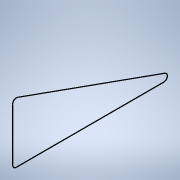
# Autodesk Inventor part: Adrian_Faden
Saved by Autodesk Inventor 2021 (Build 250183000, 183)
## iProperties
Created: 2022-07-12
Part Number: Adrian_Faden
Material: Generisch
Document SubType Name: Modeling
Designer: adria
Mass: 22.0241 g
Surface Area: 220.241 cm^2
Volume: 22.0241 cm^3
Density: 1 g/cm^3
Appearance: Vorgabe
Author: adria
Autodesk Inventor part; units mm, degrees
ref_plane "YZ Plane" through (0, 0, 0) normal (1, 0, 0) x (0, 1, 0)
ref_plane "XZ Plane" through (0, 0, 0) normal (0, 1, 0) x (-1, 0, 0)
ref_plane "XY Plane" through (0, 0, 0) normal (0, 0, 1) x (1, 0, 0)
sketch "Skizze1" plane through (0, 0, 0) normal (1, 0, 0) x (0, 1, 0)
  circle A0 centre (243.52, 0) radius 17 construction
  circle A1 centre (0, 0) radius 17 construction
  circle A2 centre (0, -680) radius 17 construction
  line L0 (243.52, 17) -> (0, 17)
  arc A3 (0, 17) -> (-17, 0) centre (0, 0) ccw
  line L1 (-17, 0) -> (-17, -680)
  arc A4 (-17, -680) -> (16.0047, -685.7316) centre (0, -680) ccw
  line L2 (16.0047, -685.7316) -> (259.5247, -5.7316)
  arc A5 (259.5247, -5.7316) -> (243.52, 17) centre (243.52, 0) ccw
  dimension "d0" = 34
  dimension "d1" = 34
  dimension "d2" = 34
  dimension "d3" = 243.52
  dimension "d4" = 680
  constraints: 6 end point, 6 point on circle, 5 centre point, 5 tangent, 2 coincident, 2 vertical alignment, 1 concentric, 1 horizontal, 1 horizontal alignment, 1 vertical, 3 other
  measures "d1" diameter of A2
  measures "d2" diameter of A0
  measures "d3" distance of point (0, 0) A0.centre
  measures "d4" distance of A2.centre point (0, 0)
sketch "Skizze2" plane through (0, 0, 0) normal (0, 0, 1) x (1, 0, 0)
  circle A0 centre (0, -17) radius 2
  line L0 (0, 243.52) -> (0, 0) projected
  point P0 (0, 0)
  point P1 (0, -17)
  dimension "d5" = 4
  constraints: 1 centre point, 1 coincident
  measures "d5" diameter of A0
sweep "Sweeping1" add profiles "Skizze2" path "Skizze1"
